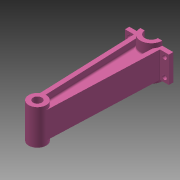
# Autodesk Inventor part: 砂轮架带动曲柄
Saved by Autodesk Inventor 2015 (Build 190159000, 159)
## iProperties
Created: 2017-05-17
Part Number: 砂轮架带动曲柄
Material: 常规
Document SubType Name: Modeling
Designer: Administrator
Density: 1 g/cm^3
Appearance: 粉红色
Author: Administrator
Autodesk Inventor part; units mm, degrees
ref_plane "YZ Plane" through (0, 0, 0) normal (1, 0, 0) x (0, 1, 0)
ref_plane "XZ Plane" through (0, 0, 0) normal (0, 1, 0) x (-1, 0, 0)
ref_plane "XY Plane" through (0, 0, 0) normal (0, 0, 1) x (1, 0, 0)
sketch "草图1" plane through (0, 0, 0) normal (0, 0, 1) x (1, 0, 0)
  arc A0 (-15, 0) -> (15, 0) centre (0, 0) ccw
  arc A1 (-7.5, 0) -> (7.5, 0) centre (0, 0) ccw
  circle A2 centre (0, -129.8) radius 10
  circle A3 centre (0, -129.8) radius 5
  line L0 (-14.9889, -0.5778) -> (-9.9926, -130.1852)
  line L1 (14.9889, -0.5778) -> (9.9926, -130.1852)
  line L2 (0, 0) -> (0, -6.0364)
  line L3 (25, 0) -> (25, -5)
  line L4 (25, -5) -> (-25, -5)
  line L5 (-25, -5) -> (-25, 0)
  line L6 (-25, 0) -> (-7.5, 0)
  line L7 (0, 0) -> (25, 0)
  line L8 (14.1421, -5) -> (25, -5)
  line L9 (25, -5) -> (25, 0)
  arc A4 (14.1421, -5) -> (15, 0) centre (0, 0) ccw
  arc A5 (-15, 0) -> (-14.1421, -5) centre (0, 0) ccw
  line L10 (-14.1421, -5) -> (-25, -5)
  line L11 (-25, 0) -> (-25, -5)
  line L12 (-25, 0) -> (-15, 0)
  dimension "d0" = 30
  dimension "d1" = 15
  dimension "d2" = 20
  dimension "d3" = 10
  dimension "d4" = 6.0365
  dimension "d5" = 129.8
  dimension "d6" = 5
  dimension "d7" = 50
  constraints: 26 end point, 14 point on circle, 6 centre point, 6 point on line, 5 collinear, 5 tangent, 4 coincident, 3 parallel, 3 perpendicular, 2 concentric, 2 horizontal, 1 vertical, 1 other
  measures "d0" diameter of A0
  measures "d1" diameter of A1
  measures "d2" diameter of A2
  measures "d3" diameter of A3
  measures "d4" distance of L2.start L2.end
  measures "d5" distance of A2.centre point (0, 0)
  measures "d6" distance of L4.end L5.end
  measures "d7" distance of L5.end L3.start
extrude "拉伸1" add sketch "草图1" along normal blind 40 contours L6 A1 L4 A0 | A0 L0 L4 L5 L6 | A0 L4 L0 | L4 A1 A0 | A0 L4 L1 A2 L0 | L4 A1 L7 A0 | A0 L1 L4 | A2 | A0 L7 L3 L4 L1
sketch "草图2" plane through (0, 0, 40) normal (0, 0, 1) x (1, 0, 0)
  line L0 (-9.7037, -7.8796) -> (-5.3299, -121.3388)
  line L1 (9.7037, -7.8796) -> (5.3299, -121.3388)
  arc A0 (-9.7037, -7.8796) -> (9.7037, -7.8796) centre (0, 0) ccw
  arc A1 (5.3299, -121.3388) -> (-5.3299, -121.3388) centre (0, -129.8) ccw
  circle A2 centre (0, -129.8) radius 5 projected
  arc A3 (-7.5, 0) -> (7.5, 0) centre (0, 0) ccw projected
  line L2 (9.9926, -130.1852) -> (14.8184, -5) projected
  line L3 (-14.8184, -5) -> (-9.9926, -130.1852) projected
  dimension "d10" = 12.5
  dimension "d11" = 10
  dimension "d12" = 5
  dimension "d13" = 5
  constraints: 4 end point, 4 point on circle, 2 centre point, 2 concentric, 2 parallel
  measures "d10" radius of A0
  measures "d11" radius of A1
  measures "d12" distance between parallel lines of L2 L1
  measures "d13" distance between parallel lines of L3 L0
extrude "拉伸2" cut sketch "草图2" against normal blind 13 contours A0 L1 A1 L0
pattern_linear "矩形阵列1" count 2 spacing 27 along (0, 0, -1) of "拉伸2"
sketch "草图3" plane through (0, 0, 40) normal (0, 0, 1) x (1, 0, 0)
  line L0 (-7.5, 0) -> (-25, 0) projected
  line L1 (25, 0) -> (7.5, 0) projected
  arc A0 (-12.5, 0) -> (12.5, 0) centre (0, 0) ccw
  arc A1 (-7.5, 0) -> (7.5, 0) centre (0, 0) ccw projected
  arc A2 (9.9926, -130.1852) -> (-9.9926, -130.1852) centre (0, -129.8) ccw
  arc A3 (-9.9926, -130.1852) -> (9.9926, -130.1852) centre (0, -129.8) ccw projected
  line L2 (9.9926, -130.1852) -> (14.8184, -5)
  line L3 (9.9926, -130.1852) -> (14.8184, -5) projected
  line L4 (14.8184, -5) -> (25, -5)
  line L5 (14.8184, -5) -> (25, -5) projected
  line L6 (25, -5) -> (25, 0)
  line L7 (25, -5) -> (25, 0) projected
  line L8 (-12.5, 0) -> (-25, 0)
  line L9 (-25, -5) -> (-14.8184, -5)
  line L10 (-14.8184, -5) -> (-9.9926, -130.1852)
  line L11 (-14.8184, -5) -> (-9.9926, -130.1852) projected
  line L12 (-25, -5) -> (-25, 0)
  line L13 (-25, 0) -> (-25, -5) projected
  dimension "d19" = 12.5
  constraints: 14 end point, 5 collinear, 4 point on circle, 2 centre point, 2 concentric, 2 horizontal, 2 point on line, 1 tangent
  measures "d19" radius of A0
extrude "拉伸3" cut sketch "草图3" against normal blind 5 contours A0 L1 L6 L4 L2 A2 L10 L9 L12 L0
pattern_linear "矩形阵列2" count 2 spacing 35 along (0, 0, -1) of "拉伸3"
sketch "草图4" plane through (-25, -5, 35) normal (0, -1, 0) x (1, 0, 0)
  circle A0 centre (5, -25) radius 2.5
  circle A1 centre (5, -5) radius 2.5
  circle A2 centre (45, -25) radius 2.5
  circle A3 centre (45, -5) radius 2.5
  line L0 (0, -30) -> (0, 0) projected
  line L1 (0, -30) -> (10.1816, -30) projected
  line L2 (10.1816, 0) -> (0, 0) projected
  line L3 (50, 0) -> (39.8184, 0) projected
  line L4 (50, -30) -> (50, 0) projected
  line L5 (39.8184, -30) -> (50, -30) projected
  point P0 (25, -35)
  dimension "d25" = 5
  dimension "d26" = 5
  dimension "d27" = 5
  dimension "d28" = 5
  dimension "d29" = 5
  dimension "d30" = 5
  dimension "d31" = 5
  dimension "d32" = 5
  dimension "d33" = 5
  dimension "d34" = 5
  dimension "d35" = 5
  dimension "d36" = 5
  constraints: 4 centre point
  measures "d25" diameter of A0
  measures "d26" diameter of A1
  measures "d27" diameter of A2
  measures "d28" diameter of A3
  measures "d29" distance from line of L0 A0.centre
  measures "d30" distance from line of L1 A0.centre
  measures "d31" distance from line of L2 A1.centre
  measures "d32" distance from line of L0 A1.centre
  measures "d33" distance from line of L3 A3.centre
  measures "d34" distance from line of L4 A3.centre
  measures "d35" distance from line of A2.centre L4
  measures "d36" distance from line of A2.centre L5
extrude "拉伸4" cut sketch "草图4" against normal through all
fillet "圆角1" radius 2 8 edges at (-7.5168, -64.6092, 13) (0, -12.5, 13) (7.5168, -64.6092, 13) (0, -119.8, 13) (0, -12.5, 27) (-7.5168, -64.6092, 27) (7.5168, -64.6092, 27) (0, -119.8, 27)
fillet "圆角2" radius 0.25 2 edges at (-14.8184, -5, 20) (14.8184, -5, 20)
